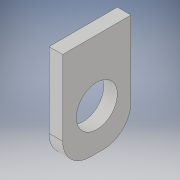
# Autodesk Inventor part: Chapa da Luz de Freio
Saved by Autodesk Inventor 2019 (Build 230136000, 136)
## iProperties
Created: 2020-06-06
Part Number: Chapa da Luz de Freio
Material: Genérico
Document SubType Name: Modeling
Designer: lukas
Density: 1 g/cm^3
Appearance: Padrão
Author: lukas
Autodesk Inventor part; units mm, degrees
ref_plane "YZ Plane" through (0, 0, 0) normal (1, 0, 0) x (0, 1, 0)
ref_plane "XZ Plane" through (0, 0, 0) normal (0, 1, 0) x (-1, 0, 0)
ref_plane "XY Plane" through (0, 0, 0) normal (0, 0, 1) x (1, 0, 0)
sketch "Esboço1" plane through (0, 0, 0) normal (1, 0, 0) x (0, 1, 0)
  line L0 (0, 0) -> (-11, 0)
  line L1 (-15, -4) -> (-15, -6)
  line L2 (-11, -10) -> (0, -10)
  line L3 (0, -10) -> (0, 0)
  arc A0 (-11, 0) -> (-15, -4) centre (-11, -4) ccw
  arc A1 (-15, -6) -> (-11, -10) centre (-11, -6) ccw
  line L4 (-15, -5) -> (-9, -5)
  circle A2 centre (-9, -5) radius 3
  point P0 (-15, -10)
  point P1 (-15, 0)
  dimension "d0" = 15
  dimension "d1" = 10
  dimension "d2" = 4
  dimension "d3" = 6
  dimension "d4" = 6
  constraints: 10 end point, 4 point on circle, 4 point on line, 4 tangent, 3 centre point, 2 horizontal, 2 parallel, 1 coincident, 1 equal radius, 1 midpoint, 1 perpendicular
  measures "d0" distance of L2.end point (-15, -10)
  measures "d1" distance of point (-15, -10) point (-15, 0)
  measures "d2" radius of A0
  measures "d3" distance of L4.start L4.end
  measures "d4" diameter of A2
extrude "Extrusão1" add sketch "Esboço1" along normal blind 2
